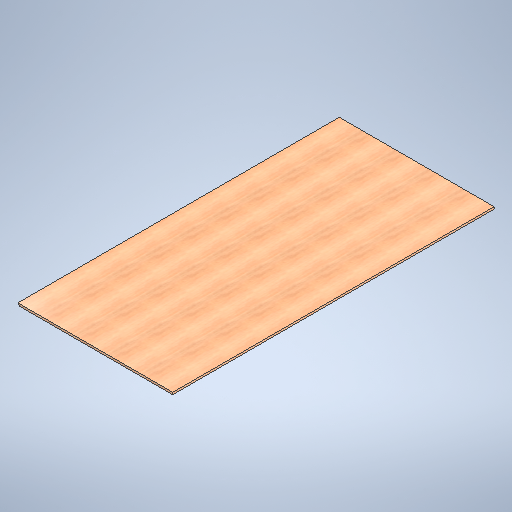
# Autodesk Inventor part: OSB_For_Roof_With_Dimensions_45.796_x_48
Saved by Autodesk Inventor 2025 (Build 290162010, 162A)
## iProperties
Created: 2024-09-17
Part Number: OSB_For_Roof_With_Dimensions_45.796_x_48
Material: Wood (Birch)
Document SubType Name: Modeling
Designer: Tom
Density: 0.55 g/cm^3
Appearance: Birch - Natural Polished
Author: Tom
Autodesk Inventor part; units mm, degrees
ref_plane "YZ Plane" through (0, 0, 0) normal (1, 0, 0) x (0, 1, 0)
ref_plane "XZ Plane" through (0, 0, 0) normal (0, 1, 0) x (-1, 0, 0)
ref_plane "XY Plane" through (0, 0, 0) normal (0, 0, 1) x (1, 0, 0)
sketch "Sketch2" plane through (0, 0, 0) normal (0, 0, 1) x (1, 0, 0)
  line L0 (0, 0) -> (-5.2225, 15.875)
  line L1 (-5.2225, 15.875) -> (1163.2184, 15.875)
  line L2 (1163.2184, 15.875) -> (1163.2184, 0)
  line L3 (1163.2184, 0) -> (0, 0)
  line L4 (0, 0) -> (0, 15.875)
  line L5 (0, 0) -> (-11.7126, 15.875)
  line L6 (-11.7126, 15.875) -> (-5.2225, 15.875)
  dimension "d7" = 1163.2184
  dimension "d8" = 15.875
  dimension "d9" = 18.21
  dimension "d10" = 18.21
  constraints: 14 end point, 3 horizontal, 2 vertical, 1 point on line
  measures "d7" distance of L2.end L0.start
  measures "d8" distance between parallel lines of L1 L3
  measures "d9" angle of L4 L0
  measures "d10" angle of L5 L0
extrude "Extrusion2" add sketch "Sketch2" along normal blind 2438.4
body "Solid2"
